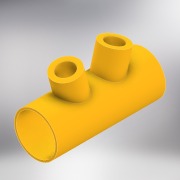
# Autodesk Inventor part: JuntaEjeCadera
Saved by Autodesk Inventor 2021 (Build 250183000, 183)
## iProperties
Created: 2024-02-21
Part Number: JuntaEjeCadera
Material: PLA
Document SubType Name: Modeling
Designer: Martin
Density: 1.27 g/cm^3
Appearance: PLA
Mass: 46.4383 g
Surface Area: 311.91 cm^2
Volume: 36.5656 cm^3
Author: Martin
Autodesk Inventor part; units mm, degrees
sketch "Sketch1" plane through (0, 0, 0) normal (0, 0, 1) x (1, 0, 0)
  circle A0 centre (0, 0) radius 18.6
  circle A1 centre (0, 0) radius 20.5
  dimension "d0" = 37.2
  dimension "d1" = 41
  constraints: 2 centre point, 2 coincident
  measures "d0" diameter of A0
  measures "d1" diameter of A1
extrude "Extrusion1" add sketch "Sketch1" along normal blind 29
ref_plane "Work Plane1" through (0, 0, 0) normal (0, 1, 0) x (0, 0, 1)
ref_plane "Work Plane2" through (0, 40.5, 0) normal (0, 1, 0) x (0, 0, 1)
sketch "Sketch3" plane through (0, 0, 29) normal (0, 0, 1) x (1, 0, 0)
  circle A0 centre (0, 0) radius 20.5 projected
  circle A1 centre (0, 0) radius 18.6 projected
extrude "Extrusion3" add sketch "Sketch3" along normal blind 22.5
ref_plane "Work Plane3" through (0, 20.5, 0) normal (0, 1, 0) x (-1, 0, 0)
sketch "Sketch5" plane through (0, 40.5, 0) normal (0, 1, 0) x (0, 0, 1)
  line L0 (0, -20.5) -> (0, 20.5) projected
  line L1 (20, 20.5) -> (20, -20.5)
  point P0 (0, 0)
  dimension "d29" = 20
  constraints: 2 end point, 1 vertical
  measures "d29" distance between parallel lines of L0 L1
ref_plane "Work Plane4" through (20.5, 40.5, 20) normal (0, 0.9659, 0.2588) x (-1, 0, 0)
sketch "Sketch8" plane through (20.5, 40.5, 20) normal (0, 0.9659, 0.2588) x (-1, 0, 0)
  circle A0 centre (20.5, 3.4439) radius 12.5
  circle A1 centre (20.5, 3.4439) radius 7.9
  point P0 (20.5, -8.8363)
  dimension "d44" = 25
  dimension "d45" = 15.8
  constraints: 2 centre point, 1 coincident
  measures "d44" diameter of A0
  measures "d45" diameter of A1
extrude "Extrusion6" add sketch "Sketch8" against normal up to surface
mirror "Mirror3" about plane through (0, 0, 0) normal (0, 0, 1) of "Extrusion1", "Extrusion6", "Extrusion3"
body "Solid1"
